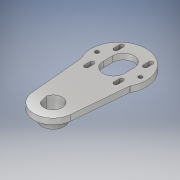
# Autodesk Inventor part: Motor Holder
Saved by Autodesk Inventor 2019.2 (Build 232265000, 265)
## iProperties
Created: 2018-12-26
Part Number: Motor Holder
Material: Aluminum 6061-AHC
Document SubType Name: Modeling
Designer: Petar
Density: 2.7 g/cm^3
Appearance: Aluminum - Dark
Author: Petar
Autodesk Inventor part; units mm, degrees
ref_plane "YZ Plane" through (0, 0, 0) normal (1, 0, 0) x (0, 1, 0)
ref_plane "XY Plane" through (0, 0, 0) normal (0, 0, 1) x (1, 0, 0)
sketch "Sketch1" plane through (0, 0, 0) normal (0, 1, 0) x (-1, 0, 0)
  line L0 (0, 58.5255) -> (0, -57.9745) construction
  line L1 (-19.918, 40.3343) -> (-25.0176, -15.8228)
  line L2 (25.0176, -15.8228) -> (19.918, 40.3343)
  arc A0 (19.918, 40.3343) -> (-19.918, 40.3343) centre (0, 38.5255) ccw
  arc A1 (-25.0176, -15.8228) -> (25.0176, -15.8228) centre (0, -29.4745) ccw
  line L3 (0, 0) -> (0, 58.5255) construction
  circle A2 centre (0, 38.5255) radius 9.5
  circle A3 centre (0, -29.4745) radius 26
  circle A4 centre (0, -29.4745) radius 21.5585 construction
  circle A5 centre (0, -29.4745) radius 22.5 construction
  circle A6 centre (-22.5, -29.4745) radius 2
  line L4 (15.2442, -44.7186) -> (-15.2442, -14.2303) construction
  line L5 (-15.2442, -44.7186) -> (15.2442, -14.2303) construction
  line L6 (15.2442, -44.7186) -> (-15.2442, -44.7186) construction
  line L7 (22.5, -29.4745) -> (-22.5, -29.4745) construction
  circle A7 centre (22.5, -29.4745) radius 2
  line L8 (-15.2442, -47.7186) -> (-15.2442, -41.7186) construction
  line L9 (-13.1442, -47.7186) -> (-13.1442, -41.7186)
  line L10 (-17.3442, -41.7186) -> (-17.3442, -47.7186)
  arc A8 (-17.3442, -47.7186) -> (-13.1442, -47.7186) centre (-15.2442, -47.7186) ccw
  arc A9 (-13.1442, -41.7186) -> (-17.3442, -41.7186) centre (-15.2442, -41.7186) ccw
  line L11 (-15.2442, -11.2303) -> (-15.2442, -17.2303) construction
  line L12 (-17.3442, -11.2303) -> (-17.3442, -17.2303)
  line L13 (-13.1442, -17.2303) -> (-13.1442, -11.2303)
  arc A10 (-13.1442, -11.2303) -> (-17.3442, -11.2303) centre (-15.2442, -11.2303) ccw
  arc A11 (-17.3442, -17.2303) -> (-13.1442, -17.2303) centre (-15.2442, -17.2303) ccw
  line L14 (-15.2442, -14.2303) -> (-9.2442, -14.2303) construction
  line L15 (15.2442, -47.7186) -> (15.2442, -41.7186) construction
  line L16 (17.3442, -47.7186) -> (17.3442, -41.7186)
  line L17 (13.1442, -41.7186) -> (13.1442, -47.7186)
  arc A12 (13.1442, -47.7186) -> (17.3442, -47.7186) centre (15.2442, -47.7186) ccw
  arc A13 (17.3442, -41.7186) -> (13.1442, -41.7186) centre (15.2442, -41.7186) ccw
  line L18 (15.2442, -44.7186) -> (21.2442, -44.7186) construction
  line L19 (15.2442, -11.2303) -> (15.2442, -17.2303) construction
  line L20 (13.1442, -11.2303) -> (13.1442, -17.2303)
  line L21 (17.3442, -17.2303) -> (17.3442, -11.2303)
  arc A14 (17.3442, -11.2303) -> (13.1442, -11.2303) centre (15.2442, -11.2303) ccw
  arc A15 (13.1442, -17.2303) -> (17.3442, -17.2303) centre (15.2442, -17.2303) ccw
  line L22 (15.2442, -14.2303) -> (21.2442, -14.2303) construction
  line L23 (0, -34.3161) -> (0, -24.3161) construction
  line L24 (11, -34.3161) -> (11, -24.3161)
  line L25 (-11, -24.3161) -> (-11, -34.3161)
  arc A16 (-11, -34.3161) -> (11, -34.3161) centre (0, -34.3161) ccw
  arc A17 (11, -24.3161) -> (-11, -24.3161) centre (0, -24.3161) ccw
  line L26 (9.1715, 36.0491) -> (6.9354, 45.0179)
  dimension "d1" = 57
  dimension "d2" = 20
  dimension "d3" = 19
  dimension "d4" = 116.5
  dimension "d5" = 68
  dimension "d6" = 52
  dimension "d8" = 43.117
  dimension "d9" = 45
  dimension "d10" = 4
  dimension "d16" = 4
  dimension "d80" = 3
  dimension "d81" = 4.2
  dimension "d82" = 3
  dimension "d83" = 90
  dimension "d84" = 4.2
  dimension "d85" = 3
  dimension "d86" = 90
  dimension "d87" = 4.2
  dimension "d88" = 3
  dimension "d89" = 90
  dimension "d90" = 4.2
  dimension "d94" = 22
  dimension "d100" = 14
  dimension "d101" = 1.2
  constraints: 64 end point, 35 point on circle, 22 tangent, 18 centre point, 7 midpoint, 7 parallel, 6 perpendicular, 6 point on line, 5 coincident, 3 horizontal, 2 vertical, 1 other
  measures "d1" diameter of A1
  measures "d2" radius of A0
  measures "d3" diameter of A2
  measures "d4" distance of L0.start L0.end
  measures "d5" distance of A0.centre A1.centre
  measures "d6" diameter of A3
  measures "d8" diameter of A4
  measures "d9" diameter of A5
  measures "d10" diameter of A6
  measures "d16" diameter of A7
  measures "d80" distance of L5.start L8.end
  measures "d81" diameter of A9
  measures "d82" distance of L4.end L11.end
  measures "d83" angle of L11 L14
  measures "d84" diameter of A11
  measures "d85" distance of L4.start L15.end
  measures "d86" angle of L18 L15
  measures "d87" diameter of A13
  measures "d88" distance of L5.end L19.end
  measures "d89" angle of L19 L22
  measures "d90" diameter of A15
  measures "d94" diameter of A17
  measures "d100" angle of L0 L26
  measures "d101" distance edge to line of A2 L26
ref_plane "Work Plane1" through (0, 3, 0) normal (0, 1, 0) x (-1, 0, 0)
sketch "Sketch2" plane through (0, 3, 0) normal (0, 1, 0) x (-1, 0, 0)
  arc A0 (-25.0176, -15.8228) -> (25.0176, -15.8228) centre (0, -29.4745) ccw projected
  line L0 (-19.918, 40.3343) -> (-25.0176, -15.8228) projected
  arc A1 (19.918, 40.3343) -> (-19.918, 40.3343) centre (0, 38.5255) ccw projected
  line L1 (25.0176, -15.8228) -> (19.918, 40.3343) projected
  circle A2 centre (0, 38.5255) radius 9.5 projected
  circle A3 centre (0, -29.4745) radius 26 projected
  circle A4 centre (15.2442, -14.0719) radius 2.1 projected
  circle A5 centre (-15.2442, -14.0719) radius 2.1 projected
  circle A6 centre (22.5, -29.4745) radius 2 projected
  circle A7 centre (-22.5, -29.4745) radius 2 projected
  circle A8 centre (-15.2442, -44.5602) radius 2.1 projected
  circle A9 centre (15.2442, -44.5602) radius 2.1 projected
  line L2 (24.6028, -11.2543) -> (10.4118, 41.3351)
  arc A10 (10.4118, 41.3351) -> (-10.3677, 41.4937) centre (0, 38.5255) ccw
  line L3 (24.6028, -11.2543) -> (-24.2003, -6.8225) construction
  line L4 (-24.2003, -6.8225) -> (-10.3677, 41.4937)
  point P0 (0, 0)
  constraints: 6 end point, 3 tangent, 2 point on circle, 2 point on line, 1 centre point, 1 coincident, 1 perpendicular
extrude "Extrusion10" add sketch "Sketch1" along normal blind 2 contours A0 L2 A1 L1 | A3
extrude "Extrusion1" add sketch "Sketch1" against normal blind 4 contours A0 L2 A1 L1 | A3 | A8 L10 A9 L9 | A10 L13 A11 L12 | A12 L17 A13 L16 | A14 L21 A15 L20 | A16 L25 A17 L24
extrude "Extrusion2" cut sketch "Sketch1" along normal through all both and the other way through all contours A2 L26 | L26 A2 | A6 | A7 | A8 L10 A9 L9 | A10 L13 A11 L12 | A12 L17 A13 L16 | A14 L21 A15 L20 | A16 L25 A17 L24
fillet "Fillet1" radius 3 2 edges at (25.0176, -1, -15.8228) (-25.0176, -1, -15.8228)
thread "Thread1" size "M4x0.7" class "6H" standard "ANSI Metric M Profile" full length
thread "Thread2" size "M4x0.7" class "6H" standard "ANSI Metric M Profile" full length
sketch "Sketch6" plane through (0, -4, 0) normal (0, -1, 0) x (1, 0, 0)
  circle A0 centre (0, 38.5255) radius 9.5 projected
  arc A1 (19.918, 40.3343) -> (-19.918, 40.3343) centre (0, 38.5255) ccw projected
  circle A2 centre (0, 38.5255) radius 11.5
  point P0 (0, 0)
  dimension "d76" = 2
  constraints: 1 centre point, 1 coincident
  measures "d76" radial gap between concentric circles of A2 A0
extrude "Extrusion6" add sketch "Sketch6" along normal blind 10
fillet "Fillet4" radius 2 1 edges at (-11.5, -4, 38.5255)
extrude "Extrusion7" cut sketch "Sketch1" along normal through all both and the other way through all contours A8 L10 A9 L9 | A10 L13 A11 L12 | A12 L17 A13 L16 | A14 L21 A15 L20
extrude "Extrusion9" add sketch "Sketch1" along normal up to surface (16 mm away) from surface at -14 contours A2 L26 picked at (8.1541, 42.3833)
body "Solid1"
